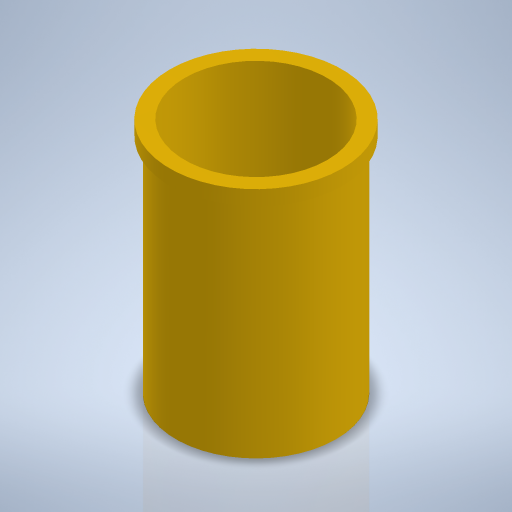
# Autodesk Inventor part: gehaeuse2
Saved by Autodesk Inventor 2024 (Build 280153000, 153)
## iProperties
Created: 2024-07-15
Part Number: gehaeuse2
Material: Blei
Document SubType Name: Modeling
Designer: ffogue
Density: 11.34 g/cm^3
Appearance: Gold
Author: ffogue
Autodesk Inventor part; units mm, degrees
ref_plane "YZ Plane" through (0, 0, 0) normal (1, 0, 0) x (0, 1, 0)
ref_plane "XZ Plane" through (0, 0, 0) normal (0, 1, 0) x (-1, 0, 0)
ref_plane "XY Plane" through (0, 0, 0) normal (0, 0, 1) x (1, 0, 0)
sketch "Skizze1" plane through (0, 0, 0) normal (0, 1, 0) x (-1, 0, 0)
  line L0 (0, 0) -> (-13.5, 0)
  line L1 (-13.5, 0) -> (-13.5, 37.5)
  line L2 (-13.5, 37.5) -> (-14.5, 37.5)
  line L3 (-14.5, 37.5) -> (-14.5, 40)
  line L4 (-14.5, 40) -> (0, 40)
  line L5 (0, 40) -> (0, 0)
  dimension "d0" = 40
  dimension "d1" = 37.5
  dimension "d2" = 29
  dimension "d3" = 27
  constraints: 12 end point, 5 perpendicular, 1 horizontal
  measures "d0" distance between parallel lines of L0 L4
  measures "d1" distance between parallel lines of L0 L2
  measures "d2" diameter of L3.end L5
  measures "d3" diameter of L1 L5
revolve "Umdrehung1" add sketch "Skizze1" angle 360 about axis through (0, 0, 40) along (0, 0, -1)
sketch "Skizze2" plane through (0, 0, 0) normal (0, 0, -1) x (-1, 0, 0)
  circle A0 centre (0, 0) radius 13.5 projected
  constraints: 1 coincident
hole "Bohrung1" at (0, 0, 0) direction (0, 0, 1) diameter 24 depth 40
